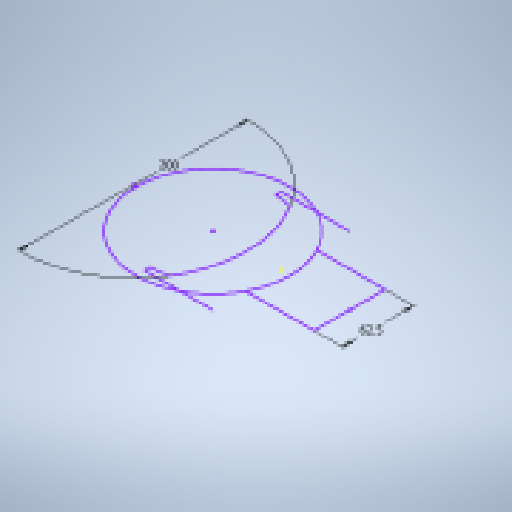
# Autodesk Inventor part: Chasis
Saved by Autodesk Inventor 2025.2 (Build 292293000, 293)
## iProperties
Created: 2025-04-24
Part Number: Chasis
Material: Genérico
Document SubType Name: Modeling
Designer: thmrc
Density: 1 g/cm^3
Appearance: Valor por defecto
Author: thmrc
Autodesk Inventor part; units mm, degrees
ref_plane "YZ Plane" through (0, 0, 0) normal (1, 0, 0) x (0, 1, 0)
ref_plane "XZ Plane" through (0, 0, 0) normal (0, 1, 0) x (-1, 0, 0)
ref_plane "XY Plane" through (0, 0, 0) normal (0, 0, 1) x (1, 0, 0)
sketch "Boceto2" plane through (0, 0, 0) normal (0, 1, 0) x (-1, 0, 0)
  line L0 (60, -60) -> (15.6267, -60)
  line L1 (15.6267, 60) -> (60, 60)
  arc A0 (45.1786, 52.9653) -> (45.1786, -52.9653) centre (130, 0) ccw
  arc A1 (45.1786, -52.9653) -> (60, -55) centre (60, 0) ccw
  arc A2 (60, 55) -> (45.1786, 52.9653) centre (60, 0) ccw
  line L2 (60, 60) -> (60, 55)
  line L3 (60, -55) -> (60, -60)
  line L4 (5, 32.5) -> (-60, 32.5)
  line L5 (5, -32.5) -> (-60, -32.5)
  line L6 (-60, -32.5) -> (-60, 32.5)
  arc A3 (15.6267, 60) -> (5, 32.5) centre (130, 0) ccw
  arc A4 (5, -32.5) -> (15.6267, -60) centre (130, 0) ccw
  line L7 (-60, 0) -> (60, 0) construction
  point P0 (0, 0)
  point P1 (30, 0)
  dimension "d8" = 200
  dimension "d13" = 65
  dimension "d17" = 65
  dimension "d18" = 65
  dimension "d19" = 30
  constraints: 16 end point, 11 point on circle, 5 centre point, 2 horizontal, 2 horizontal alignment, 1 coincident, 1 midpoint, 1 parallel, 1 vertical
  measures "d8" diameter of A0
  measures "d13" distance of L5.end L4.end
  measures "d17" distance of L4.start L4.end
  measures "d18" distance of L5.start L5.end
  measures "d19" distance of point (30, 0) L7.end
extrude "Extrusión1" add sketch "Boceto2" against normal blind 60
sketch "Boceto4" plane through (0, -60, 0) normal (0, -1, 0) x (1, 0, 0)
  line L0 (60, -32.5) -> (60, 32.5) projected
  line L1 (-5, -30) -> (60, -30)
  line L2 (60, -30) -> (60, 30)
  line L3 (60, 30) -> (-5, 30)
  line L4 (-5, 30) -> (-5, -30)
  point P0 (0, 0)
  point P1 (-5, 0)
  dimension "d22" = 60
  constraints: 8 end point, 2 parallel, 1 horizontal, 1 horizontal alignment, 1 midpoint, 1 perpendicular, 1 point on line
  measures "d22" distance of L3.end L1.start
extrude "Extrusión2" cut sketch "Boceto4" against normal blind 45
